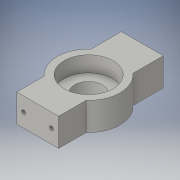
# Autodesk Inventor part: top_anchor
Saved by Autodesk Inventor 2016 (Build 200138000, 138)
## iProperties
Created: 2016-02-05
Part Number: top_anchor
Material: Generic
Document SubType Name: Modeling
Designer: Matt Ruffner
Density: 1 g/cm^3
Appearance: Default
Author: Matt Ruffner
Autodesk Inventor part; units mm, degrees
ref_plane "YZ Plane" through (0, 0, 0) normal (1, 0, 0) x (0, 1, 0)
ref_plane "XZ Plane" through (0, 0, 0) normal (0, 1, 0) x (-1, 0, 0)
ref_plane "XY Plane" through (0, 0, 0) normal (0, 0, 1) x (1, 0, 0)
sketch "Sketch1" plane through (0, 0, 0) normal (0, 1, 0) x (-1, 0, 0)
  line L0 (13.5456, 23.1663) -> (-5.5044, 23.1663)
  line L1 (-5.5044, -24.4587) -> (13.5456, -24.4587)
  line L2 (-5.5044, 23.1663) -> (-5.5044, 10.6493)
  line L3 (-5.5044, -10.6493) -> (-5.5044, -24.4587)
  line L4 (13.5456, -24.4587) -> (13.5456, -10.6493)
  line L5 (13.5456, 10.6493) -> (13.5456, 23.1663)
  circle A0 centre (4.0206, 0) radius 6.35
  arc A1 (13.5456, -10.6493) -> (13.5456, 10.6493) centre (4.0206, 0) ccw
  arc A2 (-5.5044, 10.6493) -> (-5.5044, -10.6493) centre (4.0206, 0) ccw
  point P0 (0, 0)
  dimension "d0" = 47.625
  dimension "d1" = 19.05
  dimension "d3" = 12.7
  constraints: 12 end point, 5 parallel, 4 point on circle, 3 centre point, 2 perpendicular, 1 coincident, 1 horizontal
  measures "d0" distance of L1.end L0.start
  measures "d1" distance of L0.start L0.end
  measures "d3" diameter of A0
extrude "Extrusion1" add sketch "Sketch1" along normal blind 12.7
sketch "Sketch2" plane through (0, 12.7, 0) normal (0, 1, 0) x (1, 0, 0)
  circle A0 centre (-4.0206, 0) radius 6.35 projected
  circle A1 centre (-4.0206, 0) radius 11.1125
  point P0 (0, 0)
  dimension "d7" = 22.225
  constraints: 1 centre point, 1 coincident
  measures "d7" diameter of A1
extrude "Extrusion2" cut sketch "Sketch2" against normal blind 7.112
sketch "Sketch3" plane through (-13.5456, 0, 23.1663) normal (0, 0, 1) x (1, 0, 0)
  line L0 (0, 0) -> (0, 12.7) projected
  line L1 (19.05, 0) -> (19.05, 12.7) projected
  circle A0 centre (3.175, 6.35) radius 0.889
  circle A1 centre (15.875, 6.35) radius 0.889
  point P0 (13.5456, 0)
  dimension "d10" = 3.175
  dimension "d11" = 3.175
  dimension "d12" = 1.778
  dimension "d13" = 1.778
  constraints: 2 centre point, 2 coincident
  measures "d10" distance from line of L0 point (3.175, 6.35)
  measures "d11" distance from line of L1 point (15.875, 6.35)
  measures "d12" diameter of A0
  measures "d13" diameter of A1
extrude "Extrusion3" cut sketch "Sketch3" against normal up to surface (12.5171 mm away)
sketch "Sketch4" plane through (5.5044, 0, -24.4587) normal (0, 0, -1) x (-1, 0, 0)
  circle A0 centre (3.175, 6.35) radius 0.889 projected
  circle A1 centre (15.875, 6.35) radius 0.889 projected
  point P0 (5.5044, 0)
extrude "Extrusion4" cut sketch "Sketch4" against normal up to surface (13.8094 mm away)
body "Solid1"
